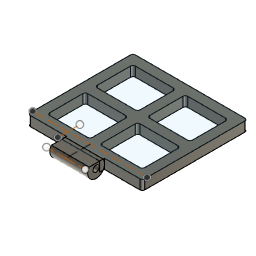
Korry_Protected_Shield (Autodesk Fusion 360 design; units mm, degrees)
Autodesk Fusion 360 part; units mm, degrees
sketch "Sketch1" plane through (0, 0, 0) normal (0, 0, 1) x (1, 0, 0)
  line L0 (0.5, 0) -> (23.2, 0)
  line L1 (23.7, 0.5) -> (23.7, 21.25)
  line L2 (23.2, 21.75) -> (0.5, 21.75)
  line L3 (0, 21.25) -> (0, 0.5)
  line L4 (23.7, 10.875) -> (0, 10.875) construction
  line L5 (11.85, 21.75) -> (11.85, 0) construction
  line L6 (10.85, 12.375) -> (10.85, 19.25)
  line L7 (10.35, 11.875) -> (2.5, 11.875)
  line L8 (10.35, 19.75) -> (2.5, 19.75)
  line L9 (2, 19.25) -> (2, 12.375)
  line L10 (13.35, 11.875) -> (21.2, 11.875)
  line L11 (12.85, 19.25) -> (12.85, 12.375)
  line L12 (21.7, 12.375) -> (21.7, 19.25)
  line L13 (21.2, 19.75) -> (13.35, 19.75)
  line L14 (12.85, 9.375) -> (12.85, 2.5)
  line L15 (13.35, 2) -> (21.2, 2)
  line L16 (21.7, 2.5) -> (21.7, 9.375)
  line L17 (21.2, 9.875) -> (13.35, 9.875)
  line L18 (10.85, 2.5) -> (10.85, 9.375)
  line L19 (2, 9.375) -> (2, 2.5)
  line L20 (2.5, 2) -> (10.35, 2)
  line L21 (10.35, 9.875) -> (2.5, 9.875)
  arc A0 (0.5, 21.75) -> (0, 21.25) centre (0.5, 21.25) ccw
  arc A1 (23.7, 21.25) -> (23.2, 21.75) centre (23.2, 21.25) ccw
  arc A2 (23.2, 0) -> (23.7, 0.5) centre (23.2, 0.5) ccw
  arc A3 (0, 0.5) -> (0.5, 0) centre (0.5, 0.5) ccw
  arc A4 (2.5, 19.75) -> (2, 19.25) centre (2.5, 19.25) ccw
  arc A5 (10.35, 11.875) -> (10.85, 12.375) centre (10.35, 12.375) ccw
  arc A6 (2, 12.375) -> (2.5, 11.875) centre (2.5, 12.375) ccw
  arc A7 (10.85, 19.25) -> (10.35, 19.75) centre (10.35, 19.25) ccw
  arc A8 (13.35, 19.75) -> (12.85, 19.25) centre (13.35, 19.25) ccw
  arc A9 (21.7, 19.25) -> (21.2, 19.75) centre (21.2, 19.25) ccw
  arc A10 (12.85, 12.375) -> (13.35, 11.875) centre (13.35, 12.375) ccw
  arc A11 (21.2, 11.875) -> (21.7, 12.375) centre (21.2, 12.375) ccw
  arc A12 (12.85, 2.5) -> (13.35, 2) centre (13.35, 2.5) ccw
  arc A13 (21.2, 2) -> (21.7, 2.5) centre (21.2, 2.5) ccw
  arc A14 (21.7, 9.375) -> (21.2, 9.875) centre (21.2, 9.375) ccw
  arc A15 (13.35, 9.875) -> (12.85, 9.375) centre (13.35, 9.375) ccw
  arc A16 (10.35, 2) -> (10.85, 2.5) centre (10.35, 2.5) ccw
  arc A17 (2, 2.5) -> (2.5, 2) centre (2.5, 2.5) ccw
  arc A18 (2.5, 9.875) -> (2, 9.375) centre (2.5, 9.375) ccw
  arc A19 (10.85, 9.375) -> (10.35, 9.875) centre (10.35, 9.375) ccw
  line L22 (11.85, 0) -> (11.85, -4)
  point P0 (10.85, 19.75)
  point P1 (10.85, 11.875)
  point P2 (2, 11.875)
  point P3 (10.85, 2)
  point P4 (2, 9.875)
  point P5 (12.85, 11.875)
  point P6 (12.85, 9.875)
  point P7 (10.85, 9.875)
  point P8 (12.85, 2)
  point P9 (21.7, 11.875)
  point P10 (21.7, 9.875)
  point P11 (12.85, 19.75)
  dimension "d1" = 23.7
  dimension "d2" = 21.75
  dimension "d14" = 0.5
  dimension "d15" = 0.5
  dimension "d16" = 0.5
  dimension "d17" = 0.5
  dimension "d18" = 0.5
  dimension "d19" = 0.5
  dimension "d20" = 0.5
  dimension "d21" = 0.5
  dimension "d22" = 0.5
  dimension "d23" = 0.5
  dimension "d24" = 0.5
  dimension "d25" = 0.5
  dimension "d26" = 0.5
  dimension "d27" = 0.5
  dimension "d28" = 0.5
  dimension "d29" = 0.5
  dimension "d30" = 0.5
  dimension "d31" = 0.5
  dimension "d32" = 0.5
  dimension "d33" = 0.5
  constraint horizontal L0
  constraint vertical L1
  constraint horizontal L2
  constraint vertical L3
  constraint perpendicular L7 L9
  constraint perpendicular L10 L11
  constraint perpendicular L10 L12
  constraint perpendicular L11 L13
  constraint perpendicular L13 L14
  constraint perpendicular L14 L15
  constraint perpendicular L13 L16
  constraint perpendicular L14 L17
  constraint perpendicular L4 L18
  constraint perpendicular L18 L20
  constraint perpendicular L18 L21
  constraint coincident L2 L5.start
  constraint coincident L3 L4.end
  constraint tangent L2 A0
  constraint tangent L3 A0
  constraint coincident L1 L4.start
  constraint tangent L1 A1
  constraint tangent L2 A1
  constraint coincident L0 L5.end
  constraint tangent L0 A2
  constraint tangent L1 A2
  constraint tangent L0 A3
  constraint tangent L3 A3
  constraint tangent L8 A4
  constraint tangent L9 A4
  constraint tangent L7 A5
  constraint tangent L6 A5
  constraint tangent L9 A6
  constraint tangent L7 A6
  constraint tangent L8 A7
  constraint tangent L6 A7
  constraint tangent L13 A8
  constraint tangent L11 A8
  constraint tangent L12 A9
  constraint tangent L13 A9
  constraint tangent L10 A10
  constraint tangent L11 A10
  constraint tangent L10 A11
  constraint tangent L12 A11
  constraint tangent L14 A12
  constraint tangent L15 A12
  constraint tangent L15 A13
  constraint tangent L16 A13
  constraint tangent L16 A14
  constraint tangent L17 A14
  constraint tangent L14 A15
  constraint tangent L17 A15
  constraint tangent L20 A16
  constraint tangent L18 A16
  constraint tangent L19 A17
  constraint tangent L20 A17
  constraint tangent L19 A18
  constraint tangent L21 A18
  constraint tangent L21 A19
  constraint tangent L18 A19
  constraint perpendicular L0 L22
  measures "d1" distance of L1 L3
  measures "d2" distance of L0 L2
  measures "d14" radius of A0
  measures "d15" radius of A1
  measures "d16" radius of A2
  measures "d17" radius of A3
  measures "d18" radius of A4
  measures "d19" radius of A5
  measures "d20" radius of A6
  measures "d21" radius of A7
  measures "d22" radius of A8
  measures "d23" radius of A9
  measures "d24" radius of A10
  measures "d25" radius of A11
  measures "d26" radius of A12
  measures "d27" radius of A13
  measures "d28" radius of A14
  measures "d29" radius of A15
  measures "d30" radius of A16
  measures "d31" radius of A17
  measures "d32" radius of A18
  measures "d33" radius of A19
extrude "Extrude1" add sketch "Sketch1" along normal blind 2 makes body 1
sketch "Sketch2" plane through (23.7, 0, 0) normal (1, 0, 0) x (0, 1, 0)
  line L0 (0.5, 0) -> (21.25, 0)
  line L1 (21.25, 0) -> (21.25, 2)
  line L2 (21.25, 2) -> (0.5, 2)
  line L3 (0.5, 2) -> (0.5, 0)
  line L4 (0.5, 1) -> (-1.7242, 1)
  circle A0 centre (-1.7242, 1) radius 1.75
  circle A1 centre (-1.7242, 1) radius 0.65
  line L5 (0, 2) -> (-3.1604, 2) construction
  line L6 (-0.2881, 2) -> (-3.1604, 2)
  line L7 (-1.7242, 1) -> (-1.6429, 1)
  point P0 (-1.6429, 1)
  dimension "d36" = 3.5
  dimension "d45" = 1.3
  constraint midpoint L3 L4.start
  constraint perpendicular L3 L4
  constraint coincident L4.end A0.centre
  constraint concentric A0 A1
  constraint coincident A0 L5.end
  constraint horizontal L5
  constraint coincident A0 L6.start
  constraint coincident L5 L6.start
  constraint parallel L4 L7
  constraint coincident P0 L7.end
  measures "d36" diameter of A0
  measures "d45" diameter of A1
extrude "Extrude2" add sketch "Sketch2" against normal blind 23.7 separate body contours A0 L6 | A0 L6 | A1 makes body 2
extrude "Extrude3" cut 1 faces at (23.7, -1.6987, 1.3838) along direction (-1, 0, 0) blind 7.85 on bodies 2 bodies 2
extrude "Extrude4" cut 1 faces at (0, -1.8298, 1.8915) along direction (1, 0, 0) blind 7.85 on bodies 2 bodies 2
sketch "Sketch3" plane through (0, 0, 2) normal (0, 0, 1) x (-1, 0, 0)
  arc A0 (-13.35, -9.875) -> (-12.85, -9.375) centre (-13.35, -9.375) ccw
  line L0 (-13.35, -9.875) -> (-21.2, -9.875)
  arc A1 (-21.7, -9.375) -> (-21.2, -9.875) centre (-21.2, -9.375) ccw
  line L1 (-21.7, -9.375) -> (-21.7, -2.5)
  arc A2 (-21.2, -2) -> (-21.7, -2.5) centre (-21.2, -2.5) ccw
  line L2 (-21.2, -2) -> (-13.35, -2)
  arc A3 (-12.85, -2.5) -> (-13.35, -2) centre (-13.35, -2.5) ccw
  line L3 (-12.85, -2.5) -> (-12.85, -9.375)
  arc A4 (-10.35, -11.875) -> (-10.85, -12.375) centre (-10.35, -12.375) ccw
  line L4 (-10.35, -11.875) -> (-2.5, -11.875)
  arc A5 (-2, -12.375) -> (-2.5, -11.875) centre (-2.5, -12.375) ccw
  line L5 (-2, -12.375) -> (-2, -19.25)
  arc A6 (-2.5, -19.75) -> (-2, -19.25) centre (-2.5, -19.25) ccw
  line L6 (-2.5, -19.75) -> (-10.35, -19.75)
  arc A7 (-10.85, -19.25) -> (-10.35, -19.75) centre (-10.35, -19.25) ccw
  line L7 (-10.85, -19.25) -> (-10.85, -12.375)
  arc A8 (-21.2, -11.875) -> (-21.7, -12.375) centre (-21.2, -12.375) ccw
  line L8 (-21.2, -11.875) -> (-13.35, -11.875)
  arc A9 (-12.85, -12.375) -> (-13.35, -11.875) centre (-13.35, -12.375) ccw
  line L9 (-12.85, -12.375) -> (-12.85, -19.25)
  arc A10 (-13.35, -19.75) -> (-12.85, -19.25) centre (-13.35, -19.25) ccw
  line L10 (-13.35, -19.75) -> (-21.2, -19.75)
  arc A11 (-21.7, -19.25) -> (-21.2, -19.75) centre (-21.2, -19.25) ccw
  line L11 (-21.7, -19.25) -> (-21.7, -12.375)
  arc A12 (-10.85, -9.375) -> (-10.35, -9.875) centre (-10.35, -9.375) ccw
  line L12 (-10.85, -9.375) -> (-10.85, -2.5)
  arc A13 (-10.35, -2) -> (-10.85, -2.5) centre (-10.35, -2.5) ccw
  line L13 (-10.35, -2) -> (-2.5, -2)
  arc A14 (-2, -2.5) -> (-2.5, -2) centre (-2.5, -2.5) ccw
  line L14 (-2, -2.5) -> (-2, -9.375)
  arc A15 (-2.5, -9.875) -> (-2, -9.375) centre (-2.5, -9.375) ccw
  line L15 (-2.5, -9.875) -> (-10.35, -9.875)
  arc A16 (0, -0.5) -> (-0.5, 0) centre (-0.5, -0.5) ccw
  line L16 (-0.5, 0) -> (-23.2, 0)
  arc A17 (-23.2, 0) -> (-23.7, -0.5) centre (-23.2, -0.5) ccw
  line L17 (-23.7, -0.5) -> (-23.7, -21.25)
  arc A18 (-23.7, -21.25) -> (-23.2, -21.75) centre (-23.2, -21.25) ccw
  line L18 (-23.2, -21.75) -> (-0.5, -21.75)
  arc A19 (-0.5, -21.75) -> (0, -21.25) centre (-0.5, -21.25) ccw
  line L19 (0, -21.25) -> (0, -0.5)
  line L20 (-23.7, -0.9888) -> (0, -0.9888) construction
  line L21 (-11.85, -0.9888) -> (-11.85, 4) construction
  line L22 (-11.85, 4) -> (-15.85, 4) construction
  line L23 (-11.85, 4) -> (-7.85, 4) construction
  dimension "d43" = 4
  dimension "d44" = 4
  constraint coincident L17 L20.start
  constraint coincident L19 L20.end
  constraint perpendicular L19 L20
  constraint midpoint L20 L21.start
  constraint perpendicular L16 L21
  constraint perpendicular L21 L22
  constraint perpendicular L21 L23
  measures "d43" distance of L21.end L22.end
  measures "d44" distance of L21.end L23.end
sketch "Sketch4" plane through (15.85, 0, 0) normal (1, 0, 0) x (0, 1, 0)
  circle A0 centre (-1.7242, 1) radius 1.75
  circle A1 centre (-1.7242, 1) radius 0.65
  dimension "d46" = 1.3
  constraint concentric A0 A1
  measures "d46" diameter of A1
extrude "Extrude5" cut sketch "Sketch4" against normal blind 8 contours A1 bodies 2
sketch "Sketch5" plane through (0, 0, 0) normal (0, -1, 0) x (1, 0, 0)
  line L0 (0.5, 0) -> (23.2, 0)
  line L1 (23.2, 0) -> (23.2, 2)
  line L2 (23.2, 2) -> (0.5, 2)
  line L3 (0.5, 2) -> (0.5, 0)
  line L4 (11.85, 2) -> (15.85, 2)
  line L5 (15.85, 2) -> (15.85, 0)
  line L6 (8, 0) -> (8, 2)
  line L7 (11.85, 2) -> (8, 2)
  line L8 (8, 0) -> (15.85, 0)
  constraint midpoint L2 L4.start
  constraint coincident L0 L5.end
  constraint perpendicular L0 L5
  constraint coincident L0 L6.start
  constraint coincident L2 L6.end
  constraint perpendicular L2 L6
  constraint perpendicular L6 L7
extrude "Extrude9" add sketch "Sketch5" along normal blind 1 contours L0 L2 L4 L5 L6 L7 L8 bodies 1
extrude "Extrude6" add sketch "Sketch5" along normal blind 2 contours L0 L2 L4 L5 L6 L7 L8 bodies 1
sketch "Sketch6" plane through (15.85, 0, 0) normal (1, 0, 0) x (0, 1, 0)
  circle A0 centre (-1.7242, 1) radius 0.65
  circle A1 centre (-1.7242, 1) radius 1.75
  line L0 (-1.6293, 2.7474) -> (-1.8191, 2.7474)
  constraint coincident A1 L0.start
  constraint coincident A1 L0.end
  constraint horizontal L0
extrude "Extrude7" cut sketch "Sketch6" against normal blind 8 contours A1 L0 picked at (-1.7137, 2.7482) bodies 2
sketch "Sketch7" plane through (0, 0, 2.7474) normal (0, 0, 1) x (-1, 0, 0)
  line L0 (-15.85, 1.8191) -> (-15.85, 1.6293)
  line L1 (-15.85, 1.6293) -> (-7.85, 1.6293)
  line L2 (-7.85, 1.6293) -> (-7.85, 1.8191)
  line L3 (-7.85, 1.8191) -> (-15.85, 1.8191)
  line L4 (-8, -2.7484) -> (-8, 1.8191) construction
  constraint coincident L3 L4.end
  constraint perpendicular L3 L4
extrude "Extrude8" cut 1 faces at (7.85, -2.9679, 0.4013) along direction (1, 0, 0) blind 0.15 on bodies 2 bodies 2
extrude "Extrude10" cut 1 faces at (10.6167, -2, 0.6667) along direction (0, 1, 0) blind 1 on bodies 1 bodies 1
sketch "Sketch9" plane through (15.85, 0, 0) normal (1, 0, 0) x (0, 1, 0)
  line L0 (-1.6293, 2.7474) -> (-1.8191, 2.7474)
  arc A0 (-1.8191, 2.7474) -> (-1.6293, 2.7474) centre (-1.7242, 1) ccw
  circle A1 centre (-1.7242, 1) radius 0.65
  line L1 (1, 2) -> (-3.1604, 2)
  constraint coincident A0 L1.end
  constraint horizontal L1
extrude "Extrude11" cut sketch "Sketch9" against normal blind 8 contours L0 A0 L1 bodies 2
